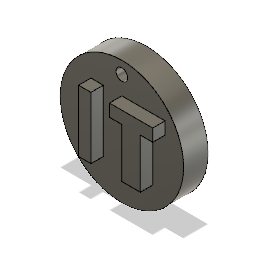
kadai1 v2 (Autodesk Fusion 360 design; units mm, degrees)
Autodesk Fusion 360 part; units mm, degrees
sketch "スケッチ1" plane through (0, 0, 0) normal (0, 0, 1) x (1, 0, 0)
  circle A0 centre (0, 0) radius 50
  constraint coincident A0.centre origin
extrude "押し出し1" add sketch "スケッチ1" along normal blind 10
sketch "スケッチ2" plane through (0, 0, 10) normal (0, 0, 1) x (1, 0, 0)
  circle A0 centre (0, 0) radius 50
  circle A1 centre (0, 40) radius 4.7499
extrude "押し出し2" cut sketch "スケッチ2" against normal blind 10 contours A1
sketch "スケッチ3" plane through (0, 0, 10) normal (0, 0, 1) x (1, 0, 0)
  circle A0 centre (0, 40) radius 4.7499
  circle A1 centre (0, 0) radius 50
sketch "スケッチ4" plane through (0, 0, 10) normal (0, 0, 1) x (1, 0, 0)
sketch "スケッチ5" plane through (0, 0, 10) normal (0, 0, 1) x (1, 0, 0)
sketch "スケッチ6" plane through (0, 0, 10) normal (0, 0, 1) x (1, 0, 0)
sketch "スケッチ7" plane through (0, 0, 10) normal (0, 0, 1) x (1, 0, 0)
sketch "スケッチ8" plane through (0, 0, 10) normal (0, 0, 1) x (1, 0, 0)
sketch "スケッチ9" plane through (0, 0, 10) normal (0, 0, 1) x (1, 0, 0)
sketch "スケッチ10" plane through (0, 0, 10) normal (0, 0, 1) x (1, 0, 0)
sketch "スケッチ11" plane through (0, 0, 10) normal (0, 0, 1) x (1, 0, 0)
sketch "スケッチ12" plane through (0, 0, 10) normal (0, 0, 1) x (1, 0, 0)
sketch "スケッチ13" plane through (0, 0, 10) normal (0, 0, 1) x (1, 0, 0)
sketch "スケッチ14" plane through (0, 0, 10) normal (0, 0, 1) x (1, 0, 0)
  line L0 (-25, 25) -> (-15, 25)
  line L1 (-15, 25) -> (-15, -30)
  line L2 (-15, -30) -> (-25, -30)
  line L3 (-25, -30) -> (-25, 25)
  line L4 (0, 25) -> (35, 25)
  line L5 (35, 25) -> (35, 15)
  line L6 (35, 15) -> (0, 15)
  line L7 (0, 15) -> (0, 25)
  line L8 (10, 15) -> (25, 15)
  line L9 (25, 15) -> (25, -30)
  line L10 (25, -30) -> (10, -30)
  line L11 (10, -30) -> (10, 15)
  constraint horizontal L0
  constraint vertical L1
  constraint horizontal L2
  constraint vertical L3
  constraint horizontal L4
  constraint vertical L5
  constraint horizontal L6
  constraint vertical L7
  constraint horizontal L8
  constraint vertical L9
  constraint horizontal L10
  constraint vertical L11
  constraint coincident L6 L8.start
extrude "押し出し3" add sketch "スケッチ14" sketch "スケッチ3" along normal blind 10 contours L0 L1 L2 L3 of sketch 2
sketch "スケッチ15" plane through (0, 0, 20) normal (0, 0, 1) x (1, 0, 0)
  circle A0 centre (0, 40) radius 4.7499
  circle A1 centre (0, 0) radius 50
  line L0 (-25, 25) -> (-15, 25)
  line L1 (-15, 25) -> (-15, -25)
  line L2 (-15, -25) -> (-25, -25)
  line L3 (-25, -25) -> (-25, 25)
  line L4 (0, 25) -> (25, 25)
  line L5 (25, 25) -> (25, 15)
  line L6 (25, 15) -> (0, 15)
  line L7 (0, 15) -> (0, 25)
  line L8 (10, 15) -> (15, 15)
  line L9 (15, 15) -> (15, -25)
  line L10 (15, -25) -> (10, -25)
  line L11 (10, -25) -> (10, 15)
  constraint horizontal L0
  constraint vertical L1
  constraint horizontal L2
  constraint vertical L3
  constraint horizontal L4
  constraint vertical L5
  constraint horizontal L6
  constraint vertical L7
  constraint horizontal L8
  constraint vertical L9
  constraint horizontal L10
  constraint vertical L11
  constraint coincident L6 L8.start
extrude "押し出し4" add sketch "スケッチ15" along normal blind 10 contours L0 L1 L2 L3
sketch "スケッチ16" plane through (0, 0, 20) normal (0, 0, 1) x (1, 0, 0)
  line L0 (-25, -25) -> (-25, 25)
  line L1 (-25, 25) -> (-15, 25)
  line L2 (-15, 25) -> (-15, -25)
  line L3 (-15, -25) -> (-25, -25)
  circle A0 centre (0, 40) radius 4.7499
  circle A1 centre (0, 0) radius 50
  line L4 (0, 25) -> (35, 25)
  line L5 (35, 25) -> (35, 15)
  line L6 (35, 15) -> (0, 15)
  line L7 (0, 15) -> (0, 25)
  line L8 (10, 15) -> (25, 15)
  line L9 (25, 15) -> (25, -25)
  line L10 (25, -25) -> (10, -25)
  line L11 (10, -25) -> (10, 15)
  constraint horizontal L4
  constraint vertical L5
  constraint horizontal L6
  constraint vertical L7
  constraint horizontal L8
  constraint vertical L9
  constraint horizontal L10
  constraint vertical L11
  constraint coincident L6 L8.start
extrude "押し出し5" add sketch "スケッチ16" along normal blind 10 contours L4 L5 L6 L7 L8 | L6 L8 L9 L10 L11
